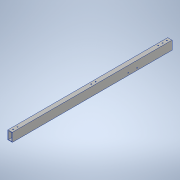
# Autodesk Inventor part: オムニ_角柱1
Saved by Autodesk Inventor 2021 (Build 250183000, 183)
## iProperties
Created: 2021-12-02
Part Number: オムニ_角柱1
Material: アルミニウム 6061
Document SubType Name: Modeling
Designer: 堀川皓史
Density: 2.7 g/cm^3
Appearance: アルミニウム - フラット
Author: 堀川皓史
Autodesk Inventor part; units mm, degrees
ref_plane "YZ Plane" through (0, 0, 0) normal (1, 0, 0) x (0, 1, 0)
ref_plane "XZ Plane" through (0, 0, 0) normal (0, 1, 0) x (-1, 0, 0)
ref_plane "XY Plane" through (0, 0, 0) normal (0, 0, 1) x (1, 0, 0)
sketch "スケッチ1" plane through (0, 0, 0) normal (0, 0, 1) x (1, 0, 0)
  line L0 (7.5, 15) -> (-7.5, 15)
  line L1 (-7.5, 15) -> (-7.5, -15)
  line L2 (-7.5, -15) -> (7.5, -15)
  line L3 (7.5, -15) -> (7.5, 15)
  line L4 (7.5, 15) -> (-7.5, -15) construction
  line L5 (-7.5, 15) -> (7.5, -15) construction
  line L6 (-5.5, 13) -> (5.5, 13)
  line L7 (5.5, 13) -> (5.5, -13)
  line L8 (5.5, -13) -> (-5.5, -13)
  line L9 (-5.5, -13) -> (-5.5, 13)
  point P0 (0, 0)
  dimension "d0" = 15
  dimension "d1" = 30
  dimension "d2" = 2
  constraints: 20 end point, 4 parallel, 2 midpoint, 2 perpendicular, 1 horizontal, 3 other
  measures "d0" distance of L2.end L1.end
  measures "d1" distance of L1.end L0.end
  measures "d2" distance between parallel lines of L0 L6
extrude "押し出し1" add sketch "スケッチ1" along normal blind 549
sketch "スケッチ2" plane through (-7.5, 15, 0) normal (0, 1, 0) x (1, 0, 0)
  circle A0 centre (7.5, -10) radius 1.6
  circle A1 centre (7.5, -25) radius 1.6
  circle A2 centre (7.5, -40) radius 1.6
  line L0 (15, 0) -> (0, 0) projected
  circle A3 centre (7.5, -255) radius 1.6
  circle A4 centre (7.5, -270) radius 1.6
  circle A5 centre (7.5, -539) radius 1.6
  circle A6 centre (7.5, -524) radius 1.6
  point P0 (7.5, 0)
  point P1 (7.5, 0)
  dimension "d5" = 3.2
  dimension "d6" = 3.2
  dimension "d7" = 3.2
  dimension "d8" = 10
  dimension "d9" = 15
  dimension "d10" = 15
  dimension "d11" = 3.2
  dimension "d12" = 3.2
  dimension "d13" = 215
  dimension "d14" = 15
  dimension "d15" = 3.2
  dimension "d16" = 3.2
  dimension "d17" = 15
  dimension "d18" = 484
  constraints: 7 centre point, 7 vertical alignment, 1 midpoint
  measures "d5" diameter of A0
  measures "d6" diameter of A1
  measures "d7" diameter of A2
  measures "d8" distance from line of L0 A0.centre
  measures "d9" distance of A0.centre A1.centre
  measures "d10" distance of A1.centre A2.centre
  measures "d11" diameter of A3
  measures "d12" diameter of A4
  measures "d13" distance of A3.centre A2.centre
  measures "d14" distance of A3.centre A4.centre
  measures "d15" diameter of A5
  measures "d16" diameter of A6
  measures "d17" distance of A6.centre A5.centre
  measures "d18" distance of A2.centre A6.centre
extrude "押し出し2" cut sketch "スケッチ2" against normal through all
sketch "スケッチ3" plane through (7.5, -15, 0) normal (1, 0, 0) x (0, 0, -1)
  circle A0 centre (-120, 7.5) radius 1.6
  circle A1 centre (-150, 7.5) radius 1.6
  line L0 (0, 0) -> (-549, 0) projected
  point P0 (0, 15)
  dimension "d21" = 3.2
  dimension "d22" = 3.2
  dimension "d23" = 30
  dimension "d24" = 7.5
  dimension "d25" = 120
  constraints: 2 centre point, 1 horizontal alignment
  measures "d21" diameter of A0
  measures "d22" diameter of A1
  measures "d23" distance of A0.centre A1.centre
  measures "d24" distance from line of L0 A0.centre
  measures "d25" horizontal distance of point (0, 15) A0.centre
extrude "押し出し3" cut sketch "スケッチ3" against normal through all
